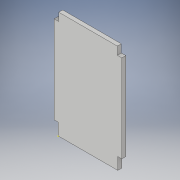
# Autodesk Inventor part: Arm Belly Pan
Saved by Autodesk Inventor 2018 (Build 220112000, 112)
## iProperties
Created: 2019-01-30
Part Number: Arm Belly Pan
Material: Generic
Document SubType Name: Modeling
Designer: maste
Density: 1 g/cm^3
Appearance: Default
Author: maste
Autodesk Inventor part; units mm, degrees
ref_plane "YZ Plane" through (0, 0, 0) normal (1, 0, 0) x (0, 1, 0)
ref_plane "XZ Plane" through (0, 0, 0) normal (0, 1, 0) x (-1, 0, 0)
ref_plane "XY Plane" through (0, 0, 0) normal (0, 0, 1) x (1, 0, 0)
sketch "Sketch1" plane through (0, 0, 0) normal (0, 0, 1) x (1, 0, 0)
  line L0 (0, 0) -> (0, 76.2)
  line L1 (0, 76.2) -> (-25.4, 76.2)
  line L2 (-25.4, 76.2) -> (-25.4, 635)
  line L3 (-25.4, 635) -> (3.175, 635)
  line L4 (3.175, 635) -> (3.175, 685.8)
  line L5 (3.175, 685.8) -> (377.825, 685.8)
  line L6 (377.825, 685.8) -> (377.825, 635)
  line L7 (377.825, 635) -> (406.4, 635)
  line L8 (406.4, 635) -> (406.4, 76.2)
  line L9 (406.4, 76.2) -> (381, 76.2)
  line L10 (381, 76.2) -> (381, 0)
  line L11 (381, 0) -> (0, 0)
  dimension "d0" = 76.2
  dimension "d1" = 25.4
  dimension "d2" = 558.8
  dimension "d3" = 28.575
  dimension "d4" = 50.8
  dimension "d5" = 374.65
  dimension "d6" = 28.575
  dimension "d7" = 25.4
  constraints: 24 end point, 9 perpendicular, 2 point on line, 2 vertical
  measures "d0" distance of L0.start L0.end
  measures "d1" distance of L0.end L1.end
  measures "d2" distance of L1.end L2.end
  measures "d3" distance of L2.end L3.end
  measures "d4" distance of L3.end L4.end
  measures "d5" distance of L4.end L5.end
  measures "d6" distance of L6.end L7.end
  measures "d7" distance of L8.end L9.end
extrude "Extrusion1" add sketch "Sketch1" along normal blind 25.4
sketch "Sketch2" plane through (0, 0, 25.4) normal (0, 0, 1) x (1, 0, 0)
  point P0 (0, 0)
body "Solid1"
